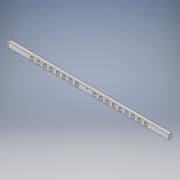
# Autodesk Inventor part: Kermit Frame 15
Saved by Autodesk Inventor 2018.2 (Build 222227000, 227)
## iProperties
Created: 2018-02-17
Part Number: Kermit Frame 15
Material: Generic
Document SubType Name: Modeling
Designer: kalra.rohan
Density: 1 g/cm^3
Appearance: Default
Author: kalra.rohan
Autodesk Inventor part; units mm, degrees
ref_plane "YZ Plane" through (0, 0, 0) normal (1, 0, 0) x (0, 1, 0)
ref_plane "XZ Plane" through (0, 0, 0) normal (0, 1, 0) x (-1, 0, 0)
ref_plane "XY Plane" through (0, 0, 0) normal (0, 0, 1) x (1, 0, 0)
sketch "Sketch1" plane through (0, 0, 0) normal (0, 0, 1) x (1, 0, 0)
  line L0 (0, 0) -> (1270, 0)
  line L1 (1270, 0) -> (1270, -38.5572)
  line L2 (1270, -38.5572) -> (0, -38.5572)
  line L3 (0, -38.5572) -> (0, 0)
  circle A0 centre (190.5, -19.2786) radius 14.0525
  circle A1 centre (241.1476, -19.2786) radius 14.0525
  circle A2 centre (291.7952, -19.2786) radius 14.0525
  circle A3 centre (342.4428, -19.2786) radius 14.0525
  circle A4 centre (393.0904, -19.2786) radius 14.0525
  circle A5 centre (443.738, -19.2786) radius 14.0525
  circle A6 centre (494.3856, -19.2786) radius 14.0525
  circle A7 centre (545.0332, -19.2786) radius 14.0525
  circle A8 centre (626.5418, -10.2743) radius 4.6546
  circle A9 centre (684.1871, -19.2786) radius 14.0526
  circle A10 centre (734.8347, -19.2786) radius 14.0526
  circle A11 centre (785.4823, -19.2786) radius 14.0526
  circle A12 centre (836.1299, -19.2786) radius 14.0526
  circle A13 centre (886.7775, -19.2786) radius 14.0526
  circle A14 centre (937.4251, -19.2786) radius 14.0526
  circle A15 centre (988.0727, -19.2786) radius 14.0526
  circle A16 centre (1038.7203, -19.2786) radius 14.0526
  circle A17 centre (1089.3679, -19.2786) radius 14.0526
  dimension "d0" = 1270
  dimension "d1" = 38.5572
  dimension "d2" = 28.1051
  dimension "d3" = 190.5
  dimension "d6" = 50.6476
  dimension "d11" = 28.2829
  dimension "d12" = 81.5086
  dimension "d13" = 9.3091
  dimension "d14" = 28.1051
  dimension "d17" = 50.6476
  dimension "d22" = 19.2786
  dimension "d23" = 19.2786
  dimension "d24" = 57.6453
  constraints: 18 centre point, 8 end point, 3 horizontal, 2 parallel, 1 perpendicular, 30 other
  measures "d0" distance between parallel lines of L1 L3
  measures "d1" distance between parallel lines of L0 L2
  measures "d2" diameter of A0
  measures "d3" distance from line of A0.centre L3
  measures "d6" distance of A0.centre A1.centre
  measures "d11" distance from line of A8.centre L2
  measures "d12" horizontal distance of A8.centre A7.centre
  measures "d13" diameter of A8
  measures "d14" diameter of A9
  measures "d17" distance of A9.centre A10.centre
  measures "d22" distance from line of L0 A0.centre
  measures "d23" distance from line of L0 A9.centre
  measures "d24" horizontal distance of A9.centre A8.centre
extrude "Extrusion1" add sketch "Sketch1" against normal blind 25.8064
sketch "Sketch2" plane through (0, 0, 0) normal (0, 0, 1) x (1, 0, 0)
  point P0 (0, 0)
body "Solid1"
